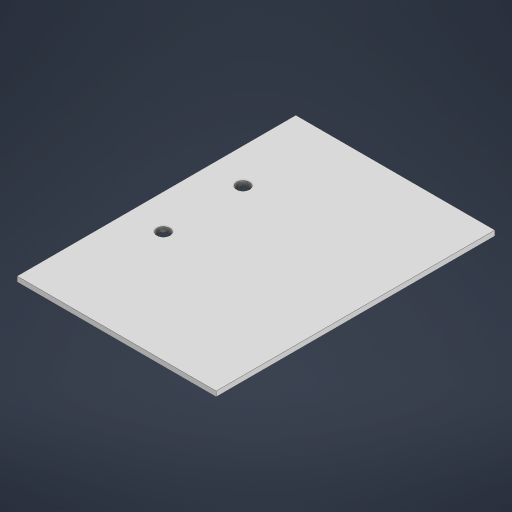
# Autodesk Inventor part: Part2
Saved by Autodesk Inventor 2023 (Build 270158000, 158)
## iProperties
Created: 2023-02-17
Part Number: Part2
Material: Generic
Document SubType Name: Modeling
Designer: Windows Macbook
Density: 1 g/cm^3
Appearance: Default
Author: Windows Macbook
Autodesk Inventor part; units mm, degrees
ref_plane "YZ Plane" through (0, 0, 0) normal (1, 0, 0) x (0, 1, 0)
ref_plane "XZ Plane" through (0, 0, 0) normal (0, 1, 0) x (-1, 0, 0)
ref_plane "XY Plane" through (0, 0, 0) normal (0, 0, 1) x (1, 0, 0)
sketch "Sketch1" plane through (0, 0, 0) normal (0, 1, 0) x (-1, 0, 0)
  line L0 (-63.5, 0) -> (-63.5, -63.5)
  line L1 (0, -63.5) -> (0, 0)
  line L2 (-63.5, 0) -> (-63.5, 17.78)
  line L3 (-63.5, 17.78) -> (0, 17.78)
  line L4 (0, 17.78) -> (0, 0)
  line L5 (-63.5, -63.5) -> (-63.5, -71.12)
  line L6 (-63.5, -71.12) -> (0, -71.12)
  line L7 (0, -71.12) -> (0, -63.5)
  dimension "d0" = 63.5
  dimension "d1" = 63.5
  dimension "d14" = 17.78
  dimension "d15" = 7.62
  constraints: 16 end point, 3 parallel
  measures "d0" distance of L1.start L0.end
  measures "d1" distance of L0.end L0.start
  measures "d14" distance of L2.start L2.end
  measures "d15" distance of L5.end L5.start
extrude "Extrusion1" add sketch "Sketch1" along normal blind 1.5875
sketch "Sketch2" plane through (0, 1.5875, 0) normal (0, 1, 0) x (1, 0, 0)
  line L0 (0, 0) -> (11.1125, 0)
  line L1 (0, 0) -> (63.5, 0) projected
  line L2 (0, 0) -> (0, 17.78)
  line L3 (0, 71.12) -> (0, 0) projected
  point P0 (0, 63.5)
  point P1 (11.1125, 17.78)
  point P2 (11.1125, 43.18)
  dimension "d4" = 11.1125
  dimension "d5" = 17.78
  constraints: 4 end point, 2 point on line
  measures "d4" distance of L0.start L0.end
  measures "d5" distance of L0.start L2.end
hole "Hole1" at (11.1125, 1.5875, -17.78) at (11.1125, 1.5875, -43.18) direction (0, -1, 0) diameter 4.1656 depth 1.5875
body "Solid1"
